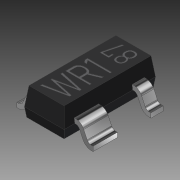
# Autodesk Inventor part: PRTR5V0U2X Protection Diode
Saved by Autodesk Inventor 2016 (Build 200138000, 138)
## iProperties
Created: 2019-08-18
Part Number: PRTR5V0U2X Protection Diode
Material: Generic
Document SubType Name: Modeling
Designer: Orest
Mass: 0.00353153 g
Surface Area: 0.19122 cm^2
Volume: 0.00353153 cm^3
Density: 1 g/cm^3
Appearance: Smooth - Black (BGA)
Catalog Web Link: https://assets.nexperia.com/documents/data-sheet/PRTR5V0U2X.pdf
Author: Orest
Autodesk Inventor part; units mm, degrees
sketch "Sketch10" plane through (0, 0, 0) normal (1, 0, 0) x (0, 1, 0)
  line L0 (-0.45, 0.65) -> (0.45, 0.65)
  line L1 (0.45, 0.65) -> (0.45, -0.65)
  line L2 (0.45, -0.65) -> (-0.45, -0.65)
  line L3 (-0.45, -0.65) -> (-0.45, 0.65)
  point P0 (0, 0)
  point P1 (0.45, 0)
  point P2 (0, 0.65)
  dimension "d7" = 0.9
  dimension "d8" = 1.3
  constraints: 8 end point, 2 midpoint, 2 parallel, 1 horizontal, 1 horizontal alignment, 1 perpendicular, 1 vertical alignment
  measures "d7" distance of L1.end L2.end
  measures "d8" distance of L0.end L1.end
extrude "Extrusion4" add sketch "Sketch10" along normal mid plane 3
chamfer "Chamfer1" distance 0.6 angle 7 1 edges at (0, 0.45, -0.65) measured on face at (-0.5, 0.15, -0.65)
chamfer "Chamfer3" distance 0.6 angle 7 1 edges at (1.5, 0.45, 0.0368) measured on face at (1.5, -0.05, 0.2167)
chamfer "Chamfer4" distance 0.6 angle 7 1 edges at (-0.0368, 0.45, 0.65) measured on face at (-0.5246, 0.15, 0.65)
chamfer "Chamfer5" distance 0.6 angle 7 1 edges at (-1.5, 0.45, 0) measured on face at (-1.5, 0.05, 0.1921)
chamfer "Chamfer2" distance 0.3 angle 7 1 edges at (0, -0.45, -0.65) measured on face at (-0.5, -0.25, -0.65)
chamfer "Chamfer6" distance 0.3 angle 7 1 edges at (1.5, -0.45, 0.0182) measured on face at (1.5, -0.2502, -0.2046)
chamfer "Chamfer7" distance 0.3 angle 7 1 edges at (-0.0182, -0.45, 0.65) measured on face at (0.4879, -0.25, 0.65)
chamfer "Chamfer8" distance 0.3 angle 7 1 edges at (-1.5, -0.45, 0) measured on face at (-1.5, -0.2503, -0.2046)
sketch "Sketch14" plane through (1.4263, 0.45, 0.5763) normal (0, 1, 0) x (1, 0, 0)
  line L0 (-2.8527, 0) -> (-2.8527, 1.1527) construction
  line L1 (0, 0) -> (-2.8527, 0) construction
  line L2 (0, 1.1527) -> (0, 0) construction
  line L3 (-2.8527, 1.1527) -> (0, 1.1527) construction
  line L4 (-2.6027, 1.0763) -> (-1.1027, 1.0763) construction
  line L5 (-1.1027, 1.0763) -> (-1.1027, 0.0763) construction
  line L6 (-1.1027, 0.0763) -> (-2.6027, 0.0763) construction
  line L7 (-2.6027, 0.0763) -> (-2.6027, 1.0763) construction
  line L8 (-0.75, 0) -> (-0.75, 1.1527) construction
  line L9 (-0.75, 1.1527) -> (-0.15, 1.1527) construction
  line L10 (-0.15, 1.1527) -> (-0.15, 0) construction
  line L11 (-0.15, 0) -> (-0.75, 0) construction
  line L12 (-2.8527, 1.1527) -> (0, 1.1527) projected
  line L13 (0, 0) -> (-2.8527, 0) projected
  line L14 (-2.3184, 0.976) -> (-2.2741, 0.976)
  line L15 (-2.2741, 0.976) -> (-2.1341, 0.2883)
  line L16 (-2.1341, 0.2883) -> (-1.9993, 0.976)
  line L17 (-1.9993, 0.976) -> (-1.928, 0.976)
  line L18 (-1.928, 0.976) -> (-2.1017, 0.176)
  line L19 (-2.1017, 0.176) -> (-2.1671, 0.176)
  line L20 (-2.1671, 0.176) -> (-2.2939, 0.8069)
  line L21 (-2.2939, 0.8069) -> (-2.4254, 0.176)
  line L22 (-2.4254, 0.176) -> (-2.4908, 0.176)
  line L23 (-2.4908, 0.176) -> (-2.6645, 0.976)
  line L24 (-2.6645, 0.976) -> (-2.5932, 0.976)
  line L25 (-2.5932, 0.976) -> (-2.4584, 0.2883)
  line L26 (-2.4584, 0.2883) -> (-2.3184, 0.976)
  line L27 (-1.7965, 0.5882) -> (-1.5778, 0.5882)
  spline S0 degree 2 poles (-1.5778, 0.5882) (-1.5428, 0.5882) (-1.4887, 0.6272) (-1.4589, 0.6985) (-1.4583, 0.7454) knots 0 0 0 1 2 3 3 3
  spline S1 degree 2 poles (-1.4583, 0.7454) (-1.4583, 0.7923) (-1.488, 0.8637) (-1.5422, 0.9027) (-1.5778, 0.9027) knots 0 0 0 1 2 3 3 3
  line L28 (-1.5778, 0.9027) -> (-1.7965, 0.9027)
  line L29 (-1.7965, 0.9027) -> (-1.7965, 0.9767)
  line L30 (-1.7965, 0.9767) -> (-1.5818, 0.9767)
  spline S2 degree 2 poles (-1.5818, 0.9767) (-1.5263, 0.9767) (-1.4424, 0.9192) (-1.3962, 0.8141) (-1.3962, 0.7454) knots 0 0 0 1 2 3 3 3
  spline S3 degree 2 poles (-1.3962, 0.7454) (-1.3962, 0.6767) (-1.4424, 0.5717) (-1.527, 0.5142) (-1.5818, 0.5142) knots 0 0 0 1 2 3 3 3
  line L31 (-1.5818, 0.5142) -> (-1.7965, 0.5142)
  line L32 (-1.7965, 0.5142) -> (-1.7965, 0.5882)
  line L33 (-1.8355, 0.9767) -> (-1.7721, 0.9767)
  line L34 (-1.7721, 0.9767) -> (-1.7721, 0.176)
  line L35 (-1.7721, 0.176) -> (-1.8355, 0.176)
  line L36 (-1.8355, 0.176) -> (-1.8355, 0.9767)
  line L37 (-1.5911, 0.5393) -> (-1.5329, 0.5644)
  line L38 (-1.5329, 0.5644) -> (-1.3691, 0.176)
  line L39 (-1.3691, 0.176) -> (-1.4451, 0.176)
  line L40 (-1.4451, 0.176) -> (-1.5911, 0.5393)
  line L41 (-1.1068, 0.176) -> (-1.1702, 0.176)
  line L42 (-1.1702, 0.176) -> (-1.1702, 0.9093)
  line L43 (-1.1702, 0.9093) -> (-1.2878, 0.8168)
  line L44 (-1.2878, 0.8168) -> (-1.2878, 0.9)
  line L45 (-1.2878, 0.9) -> (-1.1967, 0.976)
  line L46 (-1.1967, 0.976) -> (-1.1068, 0.976)
  line L47 (-1.1068, 0.976) -> (-1.1068, 0.176)
  spline S4 degree 2 poles (-0.1441, 0.3848) (-0.1441, 0.3333) (-0.1827, 0.2595) (-0.2565, 0.2208) (-0.3085, 0.2208) knots 0 0 0 1 2 3 3 3
  line L48 (-0.3085, 0.2208) -> (-0.3145, 0.2208)
  spline S5 degree 2 poles (-0.3145, 0.2208) (-0.3621, 0.2208) (-0.4379, 0.26) (-0.4597, 0.2952) knots 0 0 0 1 2 2 2
  spline S6 degree 2 poles (-0.4597, 0.2952) (-0.48, 0.2654) (-0.5483, 0.2322) (-0.5905, 0.2322) knots 0 0 0 1 2 2 2
  line L49 (-0.5905, 0.2322) -> (-0.5964, 0.2322)
  spline S7 degree 2 poles (-0.5964, 0.2322) (-0.6469, 0.2322) (-0.7188, 0.2684) (-0.7564, 0.3368) (-0.7564, 0.3848) knots 0 0 0 1 2 3 3 3
  spline S8 degree 2 poles (-0.7564, 0.3848) (-0.7564, 0.4334) (-0.7188, 0.5018) (-0.6469, 0.5374) (-0.5964, 0.5374) knots 0 0 0 1 2 3 3 3
  line L50 (-0.5964, 0.5374) -> (-0.5905, 0.5374)
  spline S9 degree 2 poles (-0.5905, 0.5374) (-0.5469, 0.5374) (-0.479, 0.5042) (-0.4597, 0.4735) knots 0 0 0 1 2 2 2
  spline S10 degree 2 poles (-0.4597, 0.4735) (-0.4379, 0.5092) (-0.3616, 0.5488) (-0.3145, 0.5488) knots 0 0 0 1 2 2 2
  line L51 (-0.3145, 0.5488) -> (-0.3085, 0.5488)
  spline S11 degree 2 poles (-0.3085, 0.5488) (-0.2565, 0.5488) (-0.1827, 0.5102) (-0.1441, 0.4364) (-0.1441, 0.3848) knots 0 0 0 1 2 3 3 3
  spline S12 degree 2 poles (-0.1981, 0.3848) (-0.1981, 0.4195) (-0.2248, 0.4681) (-0.2763, 0.4938) (-0.3125, 0.4938) knots 0 0 0 1 2 3 3 3
  line L52 (-0.3125, 0.4938) -> (-0.3145, 0.4938)
  spline S13 degree 2 poles (-0.3145, 0.4938) (-0.3507, 0.4938) (-0.4022, 0.4681) (-0.4294, 0.4195) (-0.4294, 0.3848) knots 0 0 0 1 2 3 3 3
  spline S14 degree 2 poles (-0.4294, 0.3848) (-0.4294, 0.3502) (-0.4022, 0.3016) (-0.3507, 0.2758) (-0.314, 0.2758) knots 0 0 0 1 2 3 3 3
  line L53 (-0.314, 0.2758) -> (-0.312, 0.2758)
  spline S15 degree 2 poles (-0.312, 0.2758) (-0.2758, 0.2758) (-0.2248, 0.3016) (-0.1981, 0.3502) (-0.1981, 0.3848) knots 0 0 0 1 2 3 3 3
  spline S16 degree 2 poles (-0.4815, 0.3848) (-0.4815, 0.417) (-0.5072, 0.4621) (-0.5573, 0.4859) (-0.5929, 0.4859) knots 0 0 0 1 2 3 3 3
  line L54 (-0.5929, 0.4859) -> (-0.5984, 0.4859)
  spline S17 degree 2 poles (-0.5984, 0.4859) (-0.6316, 0.4859) (-0.6777, 0.4621) (-0.7024, 0.417) (-0.7024, 0.3848) knots 0 0 0 1 2 3 3 3
  spline S18 degree 2 poles (-0.7024, 0.3848) (-0.7024, 0.3531) (-0.6777, 0.3075) (-0.6311, 0.2838) (-0.5984, 0.2838) knots 0 0 0 1 2 3 3 3
  line L55 (-0.5984, 0.2838) -> (-0.5919, 0.2838)
  spline S19 degree 2 poles (-0.5919, 0.2838) (-0.5568, 0.2838) (-0.5072, 0.3075) (-0.4815, 0.3531) (-0.4815, 0.3848) knots 0 0 0 1 2 3 3 3
  line L56 (-0.7, 0.9338) -> (-0.15, 0.7941)
  line L57 (-0.15, 0.7941) -> (-0.15, 0.7356)
  line L58 (-0.15, 0.7356) -> (-0.695, 0.8778)
  line L59 (-0.695, 0.8778) -> (-0.695, 0.6935)
  line L60 (-0.695, 0.6935) -> (-0.5835, 0.6935)
  line L61 (-0.5835, 0.6935) -> (-0.5835, 0.64)
  line L62 (-0.5835, 0.64) -> (-0.75, 0.64)
  line L63 (-0.75, 0.64) -> (-0.75, 0.9338)
  line L64 (-0.75, 0.9338) -> (-0.7, 0.9338)
  point P0 (-1.4263, 0.5763)
  point P1 (-2.6027, 0.5763)
  dimension "d53" = 0.25
  dimension "d54" = 1.5
  dimension "d55" = 1
  dimension "d56" = 0.6
  dimension "d57" = 0.15
  constraints: 2 collinear, 1 horizontal alignment, 1 midpoint, 4 other
  measures "d53" distance between parallel lines of L0 L7
  measures "d54" distance between parallel lines of L5 L7
  measures "d55" distance between parallel lines of L6 L4
  measures "d56" distance between parallel lines of L10 L8
  measures "d57" distance between parallel lines of L2 L10
extrude "Extrusion5" cut sketch "Sketch14" against normal blind 0.01 contours L14 L15 L16 L17 L18 L19 L20 L21 L22 L23 L24 L25 L26 | L32 L31 L34 L35 L36 L33 L29 L28 L27 | L27 L34 L31 L32 | L27 S0 S1 L28 L34 L30 S2 S3 L38 L37 L40 L31 | L28 L29 L30 L34 | L40 L37 L38 S3 | S3 L38 L39 L40 | L41 L42 L43 L44 L45 L46 L47 | S4 L48 S5 S6 L49 S7 S8 L50 S9 S10 L51 S11 | L56 L57 L58 L59 L60 L61 L62 L63 L64
ref_plane "Work Plane1" through (0, 0.45, 0.5763) normal (0, 0, 1) x (1, 0, 0)
sketch "Sketch11" plane through (0, 0.45, 0.5763) normal (0, 0, 1) x (1, 0, 0)
  line L0 (-1.4263, 0) -> (-1.5, -0.6) projected
  line L1 (-1.4263, 0) -> (1.4263, 0) construction
  line L2 (1.5, -0.6) -> (1.4263, 0) construction
  line L3 (1.5, -0.6) -> (-1.5, -0.6) projected
  line L4 (1.15, -0.6) -> (0.75, -0.6)
  line L5 (0.75, -0.6) -> (0.75, -0.45)
  line L6 (0.75, -0.45) -> (1.15, -0.45)
  line L7 (1.15, -0.45) -> (1.15, -0.6)
  line L8 (-0.35, -0.6) -> (-1.15, -0.6)
  line L9 (-1.15, -0.6) -> (-1.15, -0.45)
  line L10 (-1.15, -0.45) -> (-0.35, -0.45)
  line L11 (-0.35, -0.45) -> (-0.35, -0.6)
  line L12 (0, -0.6) -> (0, 0) construction
  point P0 (0, -0.45)
  dimension "d37" = 0.8
  dimension "d38" = 0.4
  dimension "d39" = 0.15
  dimension "d40" = 2.3
  constraints: 18 end point, 4 parallel, 2 collinear, 2 horizontal, 2 midpoint, 2 perpendicular, 1 point on line, 1 other
  measures "d37" distance between parallel lines of L11 L9
  measures "d38" distance between parallel lines of L7 L5
  measures "d39" distance between parallel lines of L3 L10
  measures "d40" distance between parallel lines of L7 L9
ref_plane "Work Plane2" through (1.4263, 0.45, -0.325) normal (1, 0, 0) x (0, 1, 0)
sketch "Sketch12" plane through (1.4263, 0.45, -0.325) normal (1, 0, 0) x (0, 1, 0)
  line L0 (-0.45, 0.9013) -> (-0.6, 0.9013) projected
  line L1 (-0.525, 0.9013) -> (-0.525, 0.9985)
  line L2 (-0.6549, 1.2024) -> (-0.8951, 1.3144)
  line L3 (-1.025, 1.5183) -> (-1.025, 1.575)
  line L4 (-0.9, -0.2882) -> (-0.9, 0.9382) projected
  line L5 (0, 0.9013) -> (0, -0.2513) projected
  arc A0 (-1.025, 1.5183) -> (-0.8951, 1.3144) centre (-0.8, 1.5183) ccw
  arc A1 (-0.525, 0.9985) -> (-0.6549, 1.2024) centre (-0.75, 0.9985) ccw
  line L6 (-1.025, 1.5183) -> (-1.025, 1.375) construction
  line L7 (-0.8951, 1.3144) -> (-1.025, 1.375) construction
  line L8 (0, 0.325) -> (-0.9, 0.325) construction
  line L9 (-0.45, -0.2513) -> (-0.6, -0.2513)
  line L10 (-0.525, -0.2513) -> (-0.525, -0.3485)
  line L11 (-0.6549, -0.5524) -> (-0.8951, -0.6644)
  line L12 (-1.025, -0.8683) -> (-1.025, -0.925)
  arc A2 (-0.8951, -0.6644) -> (-1.025, -0.8683) centre (-0.8, -0.8683) ccw
  arc A3 (-0.6549, -0.5524) -> (-0.525, -0.3485) centre (-0.75, -0.3485) ccw
  line L13 (-1.025, -0.8683) -> (-1.025, -0.725) construction
  line L14 (-0.8951, -0.6644) -> (-1.025, -0.725) construction
  point P0 (-0.45, 0.325)
  dimension "d42" = 1.25
  dimension "d43" = 1.025
  dimension "d45" = 0.225
  dimension "d46" = 0.2
  dimension "d47" = 65
  constraints: 24 end point, 11 symmetric about line, 8 point on circle, 6 tangent, 4 centre point, 3 midpoint, 2 parallel, 1 equal radius, 1 vertical, 2 other
  measures "d42" vertical distance of point (-0.45, 0.325) L3.end
  measures "d43" distance between parallel lines of L3 L5
  measures "d45" radius of A0
  measures "d46" distance of L6.end L3.end
  measures "d47" angle of L4 L2
ref_plane "Work Plane3" through (0, 0.45, -0.5763) normal (0, 0, -1) x (-1, 0, 0)
sketch "Sketch13" plane through (0, 0.45, -0.5763) normal (0, 0, -1) x (-1, 0, 0)
  line L0 (-1.15, -0.45) -> (-1.15, -0.6) projected
  line L1 (-0.75, -0.45) -> (-1.15, -0.45) projected
  line L2 (-0.75, -0.6) -> (-0.75, -0.45) projected
  line L3 (-1.15, -0.6) -> (-0.75, -0.6) projected
  line L4 (1.15, -0.6) -> (1.15, -0.45) projected
  line L5 (1.15, -0.45) -> (0.35, -0.45) projected
  line L6 (0.35, -0.6) -> (1.15, -0.6) projected
  line L7 (1.15, -0.45) -> (0.75, -0.45)
  line L8 (0.75, -0.45) -> (0.75, -0.6)
  line L9 (0.75, -0.6) -> (1.15, -0.6)
  line L10 (1.15, -0.6) -> (1.15, -0.45)
  point P0 (0, -0.45)
  constraints: 8 end point, 4 collinear, 2 parallel, 1 horizontal, 1 perpendicular
sweep "Sweep2" add profiles "Sketch13" path "Sketch12" path curves L10 A3 L11 A2 L12
sweep "Sweep1" add profiles "Sketch11" path "Sketch12" path curves L1 A1 L2 A0 L3
equation "\"d17\" = d11"
equation "\"d19\" = d13"
equation "\"d20\" = d11"
equation "\"d22\" = d13"
equation "\"d23\" = d11"
equation "\"d25\" = d13"
equation "\"d14\" = d7 - d11"
equation "\"d26\" = d14"
equation "\"d28\" = d16"
equation "\"d29\" = d14"
equation "\"d31\" = d16"
equation "\"d32\" = d14"
equation "\"d34\" = d16"
equation "\"d45\" = 1.5 * d39"
equation "\"d11\" = 0.6"
equation "\"d13\" = 7deg"
equation "\"d16\" = 7deg"
body "Solid4"
